Autodesk Inventor part; units mm, degrees
(part 3 of 4)
  line L1789 (3.9713, -18.6968) -> (3.9697, -18.8611)
  line L1790 (3.9697, -18.8611) -> (3.9623, -19.0574)
  line L1791 (3.9623, -19.0574) -> (3.944, -19.2862)
  line L1792 (3.944, -19.2862) -> (3.9122, -19.5462)
  line L1793 (3.9122, -19.5462) -> (3.8642, -19.8368)
  line L1794 (3.8642, -19.8368) -> (3.8334, -19.993)
  line L1795 (3.8334, -19.993) -> (3.7973, -20.1577)
  line L1796 (3.7973, -20.1577) -> (3.7564, -20.3275)
  line L1797 (3.7564, -20.3275) -> (3.709, -20.5077)
  line L1798 (3.709, -20.5077) -> (3.6602, -20.6786)
  arc A51 (2.909, -20.7975) -> (3.6602, -20.6786) centre (0, 0) ccw
  line L1799 (2.909, -20.7975) -> (2.8098, -20.6501)
  line L1800 (2.8098, -20.6501) -> (2.709, -20.4934)
  line L1801 (2.709, -20.4934) -> (2.6176, -20.3445)
  line L1802 (2.6176, -20.3445) -> (2.5324, -20.199)
  line L1803 (2.5324, -20.199) -> (2.4548, -20.06)
  line L1804 (2.4548, -20.06) -> (2.3194, -19.7984)
  line L1805 (2.3194, -19.7984) -> (2.2088, -19.561)
  line L1806 (2.2088, -19.561) -> (2.1207, -19.3491)
  line L1807 (2.1207, -19.3491) -> (2.0529, -19.1647)
  line L1808 (2.0529, -19.1647) -> (2.0007, -19.0089)
  line L1809 (2.0007, -19.0089) -> (1.9795, -18.9606)
  line L1810 (1.9795, -18.9606) -> (1.9573, -18.9216)
  line L1811 (1.9573, -18.9216) -> (1.9346, -18.8918)
  line L1812 (1.9346, -18.8918) -> (1.9116, -18.8713)
  line L1813 (1.9116, -18.8713) -> (1.8888, -18.86)
  line L1814 (1.8888, -18.86) -> (1.8665, -18.8579)
  line L1815 (1.8665, -18.8579) -> (1.833, -18.8612)
  line L1816 (1.833, -18.8612) -> (1.4868, -18.8916)
  line L1817 (1.4868, -18.8916) -> (1.1401, -18.9157)
  line L1818 (1.1401, -18.9157) -> (1.1065, -18.9177)
  line L1819 (1.1065, -18.9177) -> (1.0848, -18.9232)
  line L1820 (1.0848, -18.9232) -> (1.0641, -18.938)
  line L1821 (1.0641, -18.938) -> (1.0446, -18.9618)
  line L1822 (1.0446, -18.9618) -> (1.0268, -18.9948)
  line L1823 (1.0268, -18.9948) -> (1.011, -19.0369)
  line L1824 (1.011, -19.0369) -> (0.9976, -19.0878)
  line L1825 (0.9976, -19.0878) -> (0.9703, -19.2499)
  line L1826 (0.9703, -19.2499) -> (0.9323, -19.4427)
  line L1827 (0.9323, -19.4427) -> (0.8784, -19.6657)
  line L1828 (0.8784, -19.6657) -> (0.8063, -19.9175)
  line L1829 (0.8063, -19.9175) -> (0.7135, -20.1971)
  line L1830 (0.7135, -20.1971) -> (0.6586, -20.3465)
  line L1831 (0.6586, -20.3465) -> (0.5972, -20.5035)
  line L1832 (0.5972, -20.5035) -> (0.5302, -20.6649)
  line L1833 (0.5302, -20.6649) -> (0.4552, -20.8354)
  line L1834 (0.4552, -20.8354) -> (0.3803, -20.9966)
  arc A52 (-0.3803, -20.9966) -> (0.3803, -20.9966) centre (0, 0) ccw
  line L1835 (-0.3803, -20.9966) -> (-0.4552, -20.8354)
  line L1836 (-0.4552, -20.8354) -> (-0.5302, -20.6649)
  line L1837 (-0.5302, -20.6649) -> (-0.5972, -20.5035)
  line L1838 (-0.5972, -20.5035) -> (-0.6586, -20.3465)
  line L1839 (-0.6586, -20.3465) -> (-0.7135, -20.1971)
  line L1840 (-0.7135, -20.1971) -> (-0.8063, -19.9175)
  line L1841 (-0.8063, -19.9175) -> (-0.8784, -19.6657)
  line L1842 (-0.8784, -19.6657) -> (-0.9323, -19.4426)
  line L1843 (-0.9323, -19.4426) -> (-0.9703, -19.2499)
  line L1844 (-0.9703, -19.2499) -> (-0.9976, -19.0878)
  line L1845 (-0.9976, -19.0878) -> (-1.011, -19.0369)
  line L1846 (-1.011, -19.0369) -> (-1.0268, -18.9948)
  line L1847 (-1.0268, -18.9948) -> (-1.0446, -18.9618)
  line L1848 (-1.0446, -18.9618) -> (-1.0641, -18.938)
  line L1849 (-1.0641, -18.938) -> (-1.0848, -18.9232)
  line L1850 (-1.0848, -18.9232) -> (-1.1065, -18.9177)
  line L1851 (-1.1065, -18.9177) -> (-1.1401, -18.9157)
  line L1852 (-1.1401, -18.9157) -> (-1.4868, -18.8916)
  line L1853 (-1.4868, -18.8916) -> (-1.833, -18.8612)
  line L1854 (-1.833, -18.8612) -> (-1.8665, -18.8579)
  line L1855 (-1.8665, -18.8579) -> (-1.8888, -18.86)
  line L1856 (-1.8888, -18.86) -> (-1.9116, -18.8713)
  line L1857 (-1.9116, -18.8713) -> (-1.9346, -18.8918)
  line L1858 (-1.9346, -18.8918) -> (-1.9573, -18.9216)
  line L1859 (-1.9573, -18.9216) -> (-1.9795, -18.9606)
  line L1860 (-1.9795, -18.9606) -> (-2.0007, -19.0089)
  line L1861 (-2.0007, -19.0089) -> (-2.0529, -19.1647)
  line L1862 (-2.0529, -19.1647) -> (-2.1207, -19.3491)
  line L1863 (-2.1207, -19.3491) -> (-2.2088, -19.561)
  line L1864 (-2.2088, -19.561) -> (-2.3194, -19.7984)
  line L1865 (-2.3194, -19.7984) -> (-2.4548, -20.06)
  line L1866 (-2.4548, -20.06) -> (-2.5324, -20.199)
  line L1867 (-2.5324, -20.199) -> (-2.6176, -20.3445)
  line L1868 (-2.6176, -20.3445) -> (-2.709, -20.4934)
  line L1869 (-2.709, -20.4934) -> (-2.8098, -20.6501)
  line L1870 (-2.8098, -20.6501) -> (-2.909, -20.7975)
  arc A53 (-3.6602, -20.6786) -> (-2.909, -20.7975) centre (0, 0) ccw
  line L1871 (-3.6602, -20.6786) -> (-3.7089, -20.5077)
  line L1872 (-3.7089, -20.5077) -> (-3.7564, -20.3275)
  line L1873 (-3.7564, -20.3275) -> (-3.7973, -20.1577)
  line L1874 (-3.7973, -20.1577) -> (-3.8334, -19.993)
  line L1875 (-3.8334, -19.993) -> (-3.8642, -19.8368)
  line L1876 (-3.8642, -19.8368) -> (-3.9122, -19.5462)
  line L1877 (-3.9122, -19.5462) -> (-3.944, -19.2862)
  line L1878 (-3.944, -19.2862) -> (-3.9623, -19.0574)
  line L1879 (-3.9623, -19.0574) -> (-3.9697, -18.8611)
  line L1880 (-3.9697, -18.8611) -> (-3.9713, -18.6968)
  line L1881 (-3.9713, -18.6968) -> (-3.9765, -18.6443)
  line L1882 (-3.9765, -18.6443) -> (-3.9856, -18.6004)
  line L1883 (-3.9856, -18.6004) -> (-3.998, -18.565)
  line L1884 (-3.998, -18.565) -> (-4.0135, -18.5383)
  line L1885 (-4.0135, -18.5383) -> (-4.0317, -18.5206)
  line L1886 (-4.0317, -18.5206) -> (-4.0522, -18.5117)
  line L1887 (-4.0522, -18.5117) -> (-4.0852, -18.5045)
  line L1888 (-4.0852, -18.5045) -> (-4.4238, -18.4264)
  line L1889 (-4.4238, -18.4264) -> (-4.761, -18.3423)
  line L1890 (-4.761, -18.3423) -> (-4.7936, -18.3337)
  line L1891 (-4.7936, -18.3337) -> (-4.8159, -18.3323)
  line L1892 (-4.8159, -18.3323) -> (-4.8402, -18.3399)
  line L1893 (-4.8402, -18.3399) -> (-4.8661, -18.3566)
  line L1894 (-4.8661, -18.3566) -> (-4.8932, -18.3825)
  line L1895 (-4.8932, -18.3825) -> (-4.9212, -18.4175)
  line L1896 (-4.9212, -18.4175) -> (-4.9497, -18.4619)
  line L1897 (-4.9497, -18.4619) -> (-5.0257, -18.6076)
  line L1898 (-5.0257, -18.6076) -> (-5.1215, -18.7791)
  line L1899 (-5.1215, -18.7791) -> (-5.2416, -18.9746)
  line L1900 (-5.2416, -18.9746) -> (-5.388, -19.1919)
  line L1901 (-5.388, -19.1919) -> (-5.5627, -19.429)
  line L1902 (-5.5627, -19.429) -> (-5.661, -19.5542)
  line L1903 (-5.661, -19.5542) -> (-5.7679, -19.6846)
  line L1904 (-5.7679, -19.6846) -> (-5.8815, -19.8173)
  line L1905 (-5.8815, -19.8173) -> (-6.0056, -19.9563)
  line L1906 (-6.0056, -19.9563) -> (-6.1266, -20.0864)
  arc A54 (-6.85, -19.8514) -> (-6.1266, -20.0864) centre (0, 0) ccw
  line L1907 (-6.85, -19.8514) -> (-6.8714, -19.675)
  line L1908 (-6.8714, -19.675) -> (-6.8901, -19.4896)
  line L1909 (-6.8901, -19.4896) -> (-6.9039, -19.3155)
  line L1910 (-6.9039, -19.3155) -> (-6.9138, -19.1472)
  line L1911 (-6.9138, -19.1472) -> (-6.9198, -18.9881)
  line L1912 (-6.9198, -18.9881) -> (-6.9217, -18.6935)
  line L1913 (-6.9217, -18.6935) -> (-6.9124, -18.4318)
  line L1914 (-6.9124, -18.4318) -> (-6.8947, -18.203)
  line L1915 (-6.8947, -18.203) -> (-6.8714, -18.0079)
  line L1916 (-6.8714, -18.0079) -> (-6.8472, -17.8454)
  line L1917 (-6.8472, -17.8454) -> (-6.8442, -17.7927)
  line L1918 (-6.8442, -17.7927) -> (-6.8462, -17.7479)
  line L1919 (-6.8462, -17.7479) -> (-6.853, -17.711)
  line L1920 (-6.853, -17.711) -> (-6.8641, -17.6823)
  line L1921 (-6.8641, -17.6823) -> (-6.8793, -17.6618)
  line L1922 (-6.8793, -17.6618) -> (-6.8982, -17.6499)
  line L1923 (-6.8982, -17.6499) -> (-6.9296, -17.6376)
  line L1924 (-6.9296, -17.6376) -> (-7.2519, -17.5075)
  line L1925 (-7.2519, -17.5075) -> (-7.5717, -17.3717)
  line L1926 (-7.5717, -17.3717) -> (-7.6026, -17.3581)
  line L1927 (-7.6026, -17.3581) -> (-7.6244, -17.3532)
  line L1928 (-7.6244, -17.3532) -> (-7.6496, -17.3569)
  line L1929 (-7.6496, -17.3569) -> (-7.6778, -17.3694)
  line L1930 (-7.6778, -17.3694) -> (-7.7086, -17.3907)
  line L1931 (-7.7086, -17.3907) -> (-7.7418, -17.4209)
  line L1932 (-7.7418, -17.4209) -> (-7.7769, -17.4603)
  line L1933 (-7.7769, -17.4603) -> (-7.8747, -17.5923)
  line L1934 (-7.8747, -17.5923) -> (-7.9961, -17.7468)
  line L1935 (-7.9961, -17.7468) -> (-8.1454, -17.9211)
  line L1936 (-8.1454, -17.9211) -> (-8.3239, -18.1127)
  line L1937 (-8.3239, -18.1127) -> (-8.5336, -18.3196)
  line L1938 (-8.5336, -18.3196) -> (-8.6503, -18.4279)
  line L1939 (-8.6503, -18.4279) -> (-8.7763, -18.5399)
  line L1940 (-8.7763, -18.5399) -> (-8.9092, -18.6532)
  line L1941 (-8.9092, -18.6532) -> (-9.0535, -18.7712)
  line L1942 (-9.0535, -18.7712) -> (-9.1934, -18.8807)
  arc A55 (-9.8711, -18.5354) -> (-9.1934, -18.8807) centre (0, 0) ccw
  line L1943 (-9.8711, -18.5354) -> (-9.8647, -18.3579)
  line L1944 (-9.8647, -18.3579) -> (-9.8541, -18.1718)
  line L1945 (-9.8541, -18.1718) -> (-9.8405, -17.9977)
  line L1946 (-9.8405, -17.9977) -> (-9.8239, -17.8299)
  line L1947 (-9.8239, -17.8299) -> (-9.805, -17.6718)
  line L1948 (-9.805, -17.6718) -> (-9.7608, -17.3806)
  line L1949 (-9.7608, -17.3806) -> (-9.7107, -17.1235)
  line L1950 (-9.7107, -17.1235) -> (-9.6574, -16.9003)
  line L1951 (-9.6574, -16.9003) -> (-9.6038, -16.7112)
  line L1952 (-9.6038, -16.7112) -> (-9.5545, -16.5545)
  line L1953 (-9.5545, -16.5545) -> (-9.5433, -16.503)
  line L1954 (-9.5433, -16.503) -> (-9.5383, -16.4584)
  line L1955 (-9.5383, -16.4584) -> (-9.5392, -16.4209)
  line L1956 (-9.5392, -16.4209) -> (-9.5457, -16.3908)
  line L1957 (-9.5457, -16.3908) -> (-9.5575, -16.3682)
  line L1958 (-9.5575, -16.3682) -> (-9.5743, -16.3535)
  line L1959 (-9.5743, -16.3535) -> (-9.6034, -16.3365)
  line L1960 (-9.6034, -16.3365) -> (-9.9013, -16.1575)
  line L1961 (-9.9013, -16.1575) -> (-10.196, -15.9733)
  line L1962 (-10.196, -15.9733) -> (-10.2244, -15.9551)
  line L1963 (-10.2244, -15.9551) -> (-10.2452, -15.9469)
  line L1964 (-10.2452, -15.9469) -> (-10.2706, -15.9466)
  line L1965 (-10.2706, -15.9466) -> (-10.3004, -15.9544)
  line L1966 (-10.3004, -15.9544) -> (-10.3342, -15.9707)
  line L1967 (-10.3342, -15.9707) -> (-10.3717, -15.9954)
  line L1968 (-10.3717, -15.9954) -> (-10.4125, -16.0287)
  line L1969 (-10.4125, -16.0287) -> (-10.5298, -16.1438)
  line L1970 (-10.5298, -16.1438) -> (-10.6739, -16.2774)
  line L1971 (-10.6739, -16.2774) -> (-10.8486, -16.4262)
  line L1972 (-10.8486, -16.4262) -> (-11.0549, -16.5875)
  line L1973 (-11.0549, -16.5875) -> (-11.2943, -16.7591)
  line L1974 (-11.2943, -16.7591) -> (-11.4265, -16.8478)
  line L1975 (-11.4265, -16.8478) -> (-11.5685, -16.9387)
  line L1976 (-11.5685, -16.9387) -> (-11.7175, -17.0299)
  line L1977 (-11.7175, -17.0299) -> (-11.8785, -17.1238)
  line L1978 (-11.8785, -17.1238) -> (-12.0338, -17.2101)
  arc A56 (-12.6491, -16.7631) -> (-12.0338, -17.2101) centre (0, 0) ccw
  line L1979 (-12.6491, -16.7631) -> (-12.615, -16.5887)
  line L1980 (-12.615, -16.5887) -> (-12.5755, -16.4066)
  line L1981 (-12.5755, -16.4066) -> (-12.5348, -16.2367)
  line L1982 (-12.5348, -16.2367) -> (-12.4922, -16.0736)
  line L1983 (-12.4922, -16.0736) -> (-12.4487, -15.9204)
  line L1984 (-12.4487, -15.9204) -> (-12.3595, -15.6397)
  line L1985 (-12.3595, -15.6397) -> (-12.2698, -15.3936)
  line L1986 (-12.2698, -15.3936) -> (-12.1823, -15.1815)
  line L1987 (-12.1823, -15.1815) -> (-12.0998, -15.0031)
  line L1988 (-12.0998, -15.0031) -> (-12.0266, -14.856)
  line L1989 (-12.0266, -14.856) -> (-12.0075, -14.8069)
  line L1990 (-12.0075, -14.8069) -> (-11.9956, -14.7636)
  line L1991 (-11.9956, -14.7636) -> (-11.9906, -14.7265)
  line L1992 (-11.9906, -14.7265) -> (-11.9923, -14.6957)
  line L1993 (-11.9923, -14.6957) -> (-12.0004, -14.6716)
  line L1994 (-12.0004, -14.6716) -> (-12.0147, -14.6544)
  line L1995 (-12.0147, -14.6544) -> (-12.0408, -14.633)
  line L1996 (-12.0408, -14.633) -> (-12.307, -14.4097)
  line L1997 (-12.307, -14.4097) -> (-12.5693, -14.1816)
  line L1998 (-12.5693, -14.1816) -> (-12.5944, -14.1592)
  line L1999 (-12.5944, -14.1592) -> (-12.6137, -14.1478)
  line L2000 (-12.6137, -14.1478) -> (-12.6387, -14.1436)
  line L2001 (-12.6387, -14.1436) -> (-12.6694, -14.1467)
  line L2002 (-12.6694, -14.1467) -> (-12.7053, -14.1574)
  line L2003 (-12.7053, -14.1574) -> (-12.7462, -14.176)
  line L2004 (-12.7462, -14.176) -> (-12.7918, -14.2025)
  line L2005 (-12.7918, -14.2025) -> (-12.9256, -14.2978)
  line L2006 (-12.9256, -14.2978) -> (-13.0888, -14.4072)
  line L2007 (-13.0888, -14.4072) -> (-13.2846, -14.5269)
  line L2008 (-13.2846, -14.5269) -> (-13.5137, -14.654)
  line L2009 (-13.5137, -14.654) -> (-13.777, -14.786)
  line L2010 (-13.777, -14.786) -> (-13.9214, -14.8529)
  line L2011 (-13.9214, -14.8529) -> (-14.0759, -14.9205)
  line L2012 (-14.0759, -14.9205) -> (-14.2373, -14.9872)
  line L2013 (-14.2373, -14.9872) -> (-14.411, -15.0547)
  line L2014 (-14.411, -15.0547) -> (-14.5779, -15.1157)
  arc A57 (-15.1157, -14.5779) -> (-14.5779, -15.1157) centre (0, 0) ccw
  line L2015 (-15.1157, -14.5779) -> (-15.0547, -14.411)
  line L2016 (-15.0547, -14.411) -> (-14.9872, -14.2373)
  line L2017 (-14.9872, -14.2373) -> (-14.9205, -14.0759)
  line L2018 (-14.9205, -14.0759) -> (-14.8529, -13.9214)
  line L2019 (-14.8529, -13.9214) -> (-14.786, -13.777)
  line L2020 (-14.786, -13.777) -> (-14.654, -13.5137)
  line L2021 (-14.654, -13.5137) -> (-14.5269, -13.2846)
  line L2022 (-14.5269, -13.2846) -> (-14.4072, -13.0888)
  line L2023 (-14.4072, -13.0888) -> (-14.2978, -12.9256)
  line L2024 (-14.2978, -12.9256) -> (-14.2025, -12.7918)
  line L2025 (-14.2025, -12.7918) -> (-14.1759, -12.7462)
  line L2026 (-14.1759, -12.7462) -> (-14.1574, -12.7053)
  line L2027 (-14.1574, -12.7053) -> (-14.1467, -12.6694)
  line L2028 (-14.1467, -12.6694) -> (-14.1436, -12.6388)
  line L2029 (-14.1436, -12.6388) -> (-14.1478, -12.6137)
  line L2030 (-14.1478, -12.6137) -> (-14.1592, -12.5944)
  line L2031 (-14.1592, -12.5944) -> (-14.1816, -12.5693)
  line L2032 (-14.1816, -12.5693) -> (-14.4097, -12.307)
  line L2033 (-14.4097, -12.307) -> (-14.633, -12.0408)
  line L2034 (-14.633, -12.0408) -> (-14.6544, -12.0147)
  line L2035 (-14.6544, -12.0147) -> (-14.6716, -12.0004)
  line L2036 (-14.6716, -12.0004) -> (-14.6957, -11.9923)
  line L2037 (-14.6957, -11.9923) -> (-14.7265, -11.9906)
  line L2038 (-14.7265, -11.9906) -> (-14.7636, -11.9956)
  line L2039 (-14.7636, -11.9956) -> (-14.8069, -12.0075)
  line L2040 (-14.8069, -12.0075) -> (-14.856, -12.0266)
  line L2041 (-14.856, -12.0266) -> (-15.0031, -12.0998)
  line L2042 (-15.0031, -12.0998) -> (-15.1815, -12.1823)
  line L2043 (-15.1815, -12.1823) -> (-15.3936, -12.2699)
  line L2044 (-15.3936, -12.2699) -> (-15.6397, -12.3595)
  line L2045 (-15.6397, -12.3595) -> (-15.9204, -12.4487)
  line L2046 (-15.9204, -12.4487) -> (-16.0735, -12.4922)
  line L2047 (-16.0735, -12.4922) -> (-16.2367, -12.5348)
  line L2048 (-16.2367, -12.5348) -> (-16.4066, -12.5755)
  line L2049 (-16.4066, -12.5755) -> (-16.5887, -12.615)
  line L2050 (-16.5887, -12.615) -> (-16.763, -12.6491)
  arc A58 (-17.2101, -12.0338) -> (-16.763, -12.6491) centre (0, 0) ccw
  line L2051 (-17.2101, -12.0338) -> (-17.1238, -11.8785)
  line L2052 (-17.1238, -11.8785) -> (-17.0299, -11.7175)
  line L2053 (-17.0299, -11.7175) -> (-16.9387, -11.5685)
  line L2054 (-16.9387, -11.5685) -> (-16.8478, -11.4266)
  line L2055 (-16.8478, -11.4266) -> (-16.7591, -11.2943)
  line L2056 (-16.7591, -11.2943) -> (-16.5875, -11.0549)
  line L2057 (-16.5875, -11.0549) -> (-16.4262, -10.8486)
  line L2058 (-16.4262, -10.8486) -> (-16.2774, -10.6739)
  line L2059 (-16.2774, -10.6739) -> (-16.1438, -10.5298)
  line L2060 (-16.1438, -10.5298) -> (-16.0287, -10.4125)
  line L2061 (-16.0287, -10.4125) -> (-15.9954, -10.3717)
  line L2062 (-15.9954, -10.3717) -> (-15.9707, -10.3342)
  line L2063 (-15.9707, -10.3342) -> (-15.9544, -10.3004)
  line L2064 (-15.9544, -10.3004) -> (-15.9466, -10.2706)
  line L2065 (-15.9466, -10.2706) -> (-15.9468, -10.2452)
  line L2066 (-15.9468, -10.2452) -> (-15.9551, -10.2244)
  line L2067 (-15.9551, -10.2244) -> (-15.9733, -10.196)
  line L2068 (-15.9733, -10.196) -> (-16.1575, -9.9014)
  line L2069 (-16.1575, -9.9014) -> (-16.3364, -9.6034)
  line L2070 (-16.3364, -9.6034) -> (-16.3534, -9.5743)
  line L2071 (-16.3534, -9.5743) -> (-16.3682, -9.5575)
  line L2072 (-16.3682, -9.5575) -> (-16.3908, -9.5457)
  line L2073 (-16.3908, -9.5457) -> (-16.4209, -9.5392)
  line L2074 (-16.4209, -9.5392) -> (-16.4584, -9.5383)
  line L2075 (-16.4584, -9.5383) -> (-16.503, -9.5433)
  line L2076 (-16.503, -9.5433) -> (-16.5545, -9.5545)
  line L2077 (-16.5545, -9.5545) -> (-16.7112, -9.6038)
  line L2078 (-16.7112, -9.6038) -> (-16.9003, -9.6574)
  line L2079 (-16.9003, -9.6574) -> (-17.1235, -9.7107)
  line L2080 (-17.1235, -9.7107) -> (-17.3806, -9.7608)
  line L2081 (-17.3806, -9.7608) -> (-17.6718, -9.805)
  line L2082 (-17.6718, -9.805) -> (-17.8299, -9.8239)
  line L2083 (-17.8299, -9.8239) -> (-17.9976, -9.8405)
  line L2084 (-17.9976, -9.8405) -> (-18.1718, -9.8541)
  line L2085 (-18.1718, -9.8541) -> (-18.3579, -9.8647)
  line L2086 (-18.3579, -9.8647) -> (-18.5354, -9.8711)
  arc A59 (-18.8807, -9.1934) -> (-18.5354, -9.8711) centre (0, 0) ccw
  line L2087 (-18.8807, -9.1934) -> (-18.7712, -9.0535)
  line L2088 (-18.7712, -9.0535) -> (-18.6532, -8.9092)
  line L2089 (-18.6532, -8.9092) -> (-18.5399, -8.7763)
  line L2090 (-18.5399, -8.7763) -> (-18.4279, -8.6503)
  line L2091 (-18.4279, -8.6503) -> (-18.3196, -8.5336)
  line L2092 (-18.3196, -8.5336) -> (-18.1127, -8.324)
  line L2093 (-18.1127, -8.324) -> (-17.9211, -8.1454)
  line L2094 (-17.9211, -8.1454) -> (-17.7468, -7.9961)
  line L2095 (-17.7468, -7.9961) -> (-17.5923, -7.8747)
  line L2096 (-17.5923, -7.8747) -> (-17.4603, -7.7769)
  line L2097 (-17.4603, -7.7769) -> (-17.4209, -7.7418)
  line L2098 (-17.4209, -7.7418) -> (-17.3907, -7.7086)
  line L2099 (-17.3907, -7.7086) -> (-17.3694, -7.6778)
  line L2100 (-17.3694, -7.6778) -> (-17.3569, -7.6496)
  line L2101 (-17.3569, -7.6496) -> (-17.3532, -7.6244)
  line L2102 (-17.3532, -7.6244) -> (-17.3581, -7.6026)
  line L2103 (-17.3581, -7.6026) -> (-17.3717, -7.5717)
  line L2104 (-17.3717, -7.5717) -> (-17.5075, -7.2519)
  line L2105 (-17.5075, -7.2519) -> (-17.6376, -6.9296)
  line L2106 (-17.6376, -6.9296) -> (-17.6499, -6.8982)
  line L2107 (-17.6499, -6.8982) -> (-17.6618, -6.8793)
  line L2108 (-17.6618, -6.8793) -> (-17.6823, -6.8641)
  line L2109 (-17.6823, -6.8641) -> (-17.711, -6.853)
  line L2110 (-17.711, -6.853) -> (-17.7479, -6.8462)
  line L2111 (-17.7479, -6.8462) -> (-17.7927, -6.8442)
  line L2112 (-17.7927, -6.8442) -> (-17.8453, -6.8472)
  line L2113 (-17.8453, -6.8472) -> (-18.0079, -6.8714)
  line L2114 (-18.0079, -6.8714) -> (-18.203, -6.8948)
  line L2115 (-18.203, -6.8948) -> (-18.4318, -6.9124)
  line L2116 (-18.4318, -6.9124) -> (-18.6935, -6.9217)
  line L2117 (-18.6935, -6.9217) -> (-18.9881, -6.9198)
  line L2118 (-18.9881, -6.9198) -> (-19.1471, -6.9138)
  line L2119 (-19.1471, -6.9138) -> (-19.3155, -6.9039)
  line L2120 (-19.3155, -6.9039) -> (-19.4896, -6.8901)
  line L2121 (-19.4896, -6.8901) -> (-19.675, -6.8714)
  line L2122 (-19.675, -6.8714) -> (-19.8514, -6.85)
  arc A60 (-20.0864, -6.1266) -> (-19.8514, -6.85) centre (0, 0) ccw
  line L2123 (-20.0864, -6.1266) -> (-19.9563, -6.0056)
  line L2124 (-19.9563, -6.0056) -> (-19.8173, -5.8815)
  line L2125 (-19.8173, -5.8815) -> (-19.6846, -5.768)
  line L2126 (-19.6846, -5.768) -> (-19.5542, -5.661)
  line L2127 (-19.5542, -5.661) -> (-19.429, -5.5627)
  line L2128 (-19.429, -5.5627) -> (-19.1918, -5.388)
  line L2129 (-19.1918, -5.388) -> (-18.9746, -5.2416)
  line L2130 (-18.9746, -5.2416) -> (-18.7791, -5.1215)
  line L2131 (-18.7791, -5.1215) -> (-18.6076, -5.0257)
  line L2132 (-18.6076, -5.0257) -> (-18.4619, -4.9497)
  line L2133 (-18.4619, -4.9497) -> (-18.4175, -4.9212)
  line L2134 (-18.4175, -4.9212) -> (-18.3824, -4.8932)
  line L2135 (-18.3824, -4.8932) -> (-18.3566, -4.8661)
  line L2136 (-18.3566, -4.8661) -> (-18.3399, -4.8402)
  line L2137 (-18.3399, -4.8402) -> (-18.3323, -4.8159)
  line L2138 (-18.3323, -4.8159) -> (-18.3337, -4.7936)
  line L2139 (-18.3337, -4.7936) -> (-18.3423, -4.761)
  line L2140 (-18.3423, -4.761) -> (-18.4264, -4.4238)
  line L2141 (-18.4264, -4.4238) -> (-18.5045, -4.0852)
  line L2142 (-18.5045, -4.0852) -> (-18.5117, -4.0522)
  line L2143 (-18.5117, -4.0522) -> (-18.5205, -4.0317)
  line L2144 (-18.5205, -4.0317) -> (-18.5383, -4.0135)
  line L2145 (-18.5383, -4.0135) -> (-18.565, -3.998)
  line L2146 (-18.565, -3.998) -> (-18.6003, -3.9856)
  line L2147 (-18.6003, -3.9856) -> (-18.6443, -3.9765)
  line L2148 (-18.6443, -3.9765) -> (-18.6968, -3.9713)
  line L2149 (-18.6968, -3.9713) -> (-18.8611, -3.9697)
  line L2150 (-18.8611, -3.9697) -> (-19.0574, -3.9623)
  line L2151 (-19.0574, -3.9623) -> (-19.2862, -3.944)
  line L2152 (-19.2862, -3.944) -> (-19.5462, -3.9122)
  line L2153 (-19.5462, -3.9122) -> (-19.8368, -3.8642)
  line L2154 (-19.8368, -3.8642) -> (-19.993, -3.8334)
  line L2155 (-19.993, -3.8334) -> (-20.1577, -3.7973)
  line L2156 (-20.1577, -3.7973) -> (-20.3275, -3.7564)
  line L2157 (-20.3275, -3.7564) -> (-20.5077, -3.709)
  line L2158 (-20.5077, -3.709) -> (-20.6786, -3.6602)
  arc A61 (-20.7975, -2.909) -> (-20.6786, -3.6602) centre (0, 0) ccw
  line L2159 (-20.7975, -2.909) -> (-20.6501, -2.8098)
  line L2160 (-20.6501, -2.8098) -> (-20.4934, -2.709)
  line L2161 (-20.4934, -2.709) -> (-20.3445, -2.6176)
  line L2162 (-20.3445, -2.6176) -> (-20.199, -2.5324)
  line L2163 (-20.199, -2.5324) -> (-20.06, -2.4549)
  line L2164 (-20.06, -2.4549) -> (-19.7984, -2.3194)
  line L2165 (-19.7984, -2.3194) -> (-19.561, -2.2088)
  line L2166 (-19.561, -2.2088) -> (-19.3491, -2.1207)
  line L2167 (-19.3491, -2.1207) -> (-19.1647, -2.053)
  line L2168 (-19.1647, -2.053) -> (-19.0089, -2.0007)
  line L2169 (-19.0089, -2.0007) -> (-18.9606, -1.9795)
  line L2170 (-18.9606, -1.9795) -> (-18.9216, -1.9573)
  line L2171 (-18.9216, -1.9573) -> (-18.8918, -1.9346)
  line L2172 (-18.8918, -1.9346) -> (-18.8713, -1.9116)
  line L2173 (-18.8713, -1.9116) -> (-18.8599, -1.8888)
  line L2174 (-18.8599, -1.8888) -> (-18.8579, -1.8665)
  line L2175 (-18.8579, -1.8665) -> (-18.8612, -1.833)
  line L2176 (-18.8612, -1.833) -> (-18.8916, -1.4868)
  line L2177 (-18.8916, -1.4868) -> (-18.9157, -1.1401)
  line L2178 (-18.9157, -1.1401) -> (-18.9177, -1.1065)
  line L2179 (-18.9177, -1.1065) -> (-18.9232, -1.0848)
  line L2180 (-18.9232, -1.0848) -> (-18.938, -1.0641)
  line L2181 (-18.938, -1.0641) -> (-18.9618, -1.0446)
  line L2182 (-18.9618, -1.0446) -> (-18.9948, -1.0268)
  line L2183 (-18.9948, -1.0268) -> (-19.0368, -1.011)
  line L2184 (-19.0368, -1.011) -> (-19.0878, -0.9976)
  line L2185 (-19.0878, -0.9976) -> (-19.2499, -0.9703)
  line L2186 (-19.2499, -0.9703) -> (-19.4426, -0.9323)
  line L2187 (-19.4426, -0.9323) -> (-19.6657, -0.8784)
  line L2188 (-19.6657, -0.8784) -> (-19.9175, -0.8063)
  line L2189 (-19.9175, -0.8063) -> (-20.1971, -0.7135)
  line L2190 (-20.1971, -0.7135) -> (-20.3465, -0.6586)
  line L2191 (-20.3465, -0.6586) -> (-20.5035, -0.5972)
  line L2192 (-20.5035, -0.5972) -> (-20.6649, -0.5302)
  line L2193 (-20.6649, -0.5302) -> (-20.8354, -0.4552)
  line L2194 (-20.8354, -0.4552) -> (-20.9966, -0.3803)
  arc A62 (-20.9966, 0.3803) -> (-20.9966, -0.3803) centre (0, 0) ccw
  line L2195 (-20.9966, 0.3803) -> (-20.8354, 0.4552)
  line L2196 (-20.8354, 0.4552) -> (-20.6649, 0.5302)
  line L2197 (-20.6649, 0.5302) -> (-20.5035, 0.5972)
  line L2198 (-20.5035, 0.5972) -> (-20.3465, 0.6586)
  line L2199 (-20.3465, 0.6586) -> (-20.1971, 0.7134)
  line L2200 (-20.1971, 0.7134) -> (-19.9175, 0.8063)
  line L2201 (-19.9175, 0.8063) -> (-19.6657, 0.8784)
  line L2202 (-19.6657, 0.8784) -> (-19.4426, 0.9323)
  line L2203 (-19.4426, 0.9323) -> (-19.2499, 0.9703)
  line L2204 (-19.2499, 0.9703) -> (-19.0878, 0.9976)
  line L2205 (-19.0878, 0.9976) -> (-19.0368, 1.011)
  line L2206 (-19.0368, 1.011) -> (-18.9948, 1.0268)
  line L2207 (-18.9948, 1.0268) -> (-18.9618, 1.0446)
  line L2208 (-18.9618, 1.0446) -> (-18.938, 1.0641)
  line L2209 (-18.938, 1.0641) -> (-18.9232, 1.0848)
  line L2210 (-18.9232, 1.0848) -> (-18.9177, 1.1065)
  line L2211 (-18.9177, 1.1065) -> (-18.9157, 1.1401)
  line L2212 (-18.9157, 1.1401) -> (-18.8916, 1.4868)
  line L2213 (-18.8916, 1.4868) -> (-18.8612, 1.833)
  line L2214 (-18.8612, 1.833) -> (-18.8579, 1.8665)
  line L2215 (-18.8579, 1.8665) -> (-18.8599, 1.8888)
  line L2216 (-18.8599, 1.8888) -> (-18.8713, 1.9116)
  line L2217 (-18.8713, 1.9116) -> (-18.8918, 1.9346)
  line L2218 (-18.8918, 1.9346) -> (-18.9216, 1.9573)
  line L2219 (-18.9216, 1.9573) -> (-18.9606, 1.9795)
  line L2220 (-18.9606, 1.9795) -> (-19.0089, 2.0007)
  line L2221 (-19.0089, 2.0007) -> (-19.1647, 2.0529)
  line L2222 (-19.1647, 2.0529) -> (-19.3491, 2.1207)
  line L2223 (-19.3491, 2.1207) -> (-19.561, 2.2088)
  line L2224 (-19.561, 2.2088) -> (-19.7984, 2.3194)
  line L2225 (-19.7984, 2.3194) -> (-20.06, 2.4548)
  line L2226 (-20.06, 2.4548) -> (-20.199, 2.5324)
  line L2227 (-20.199, 2.5324) -> (-20.3445, 2.6176)
  line L2228 (-20.3445, 2.6176) -> (-20.4934, 2.709)
  line L2229 (-20.4934, 2.709) -> (-20.6501, 2.8098)
  line L2230 (-20.6501, 2.8098) -> (-20.7975, 2.909)
  arc A63 (-20.6786, 3.6602) -> (-20.7975, 2.909) centre (0, 0) ccw
  line L2231 (-20.6786, 3.6602) -> (-20.5077, 3.7089)
  line L2232 (-20.5077, 3.7089) -> (-20.3275, 3.7564)
  line L2233 (-20.3275, 3.7564) -> (-20.1577, 3.7973)
  line L2234 (-20.1577, 3.7973) -> (-19.993, 3.8334)
  line L2235 (-19.993, 3.8334) -> (-19.8368, 3.8642)
  line L2236 (-19.8368, 3.8642) -> (-19.5462, 3.9121)
  line L2237 (-19.5462, 3.9121) -> (-19.2862, 3.944)
  line L2238 (-19.2862, 3.944) -> (-19.0574, 3.9623)
  line L2239 (-19.0574, 3.9623) -> (-18.8611, 3.9697)
  line L2240 (-18.8611, 3.9697) -> (-18.6968, 3.9713)
  line L2241 (-18.6968, 3.9713) -> (-18.6443, 3.9765)
  line L2242 (-18.6443, 3.9765) -> (-18.6003, 3.9856)
  line L2243 (-18.6003, 3.9856) -> (-18.565, 3.998)
  line L2244 (-18.565, 3.998) -> (-18.5383, 4.0135)
  line L2245 (-18.5383, 4.0135) -> (-18.5205, 4.0317)
  line L2246 (-18.5205, 4.0317) -> (-18.5117, 4.0522)
  line L2247 (-18.5117, 4.0522) -> (-18.5045, 4.0851)
  line L2248 (-18.5045, 4.0851) -> (-18.4264, 4.4238)
  line L2249 (-18.4264, 4.4238) -> (-18.3423, 4.761)
  line L2250 (-18.3423, 4.761) -> (-18.3337, 4.7936)
  line L2251 (-18.3337, 4.7936) -> (-18.3323, 4.8159)
  line L2252 (-18.3323, 4.8159) -> (-18.3399, 4.8402)
  line L2253 (-18.3399, 4.8402) -> (-18.3566, 4.8661)
  line L2254 (-18.3566, 4.8661) -> (-18.3824, 4.8932)
  line L2255 (-18.3824, 4.8932) -> (-18.4175, 4.9212)
  line L2256 (-18.4175, 4.9212) -> (-18.4619, 4.9497)
  line L2257 (-18.4619, 4.9497) -> (-18.6076, 5.0257)
  line L2258 (-18.6076, 5.0257) -> (-18.7791, 5.1215)
  line L2259 (-18.7791, 5.1215) -> (-18.9746, 5.2416)
  line L2260 (-18.9746, 5.2416) -> (-19.1918, 5.388)
  line L2261 (-19.1918, 5.388) -> (-19.429, 5.5627)
  line L2262 (-19.429, 5.5627) -> (-19.5542, 5.661)
  line L2263 (-19.5542, 5.661) -> (-19.6846, 5.7679)
  line L2264 (-19.6846, 5.7679) -> (-19.8173, 5.8815)
  line L2265 (-19.8173, 5.8815) -> (-19.9563, 6.0056)
  line L2266 (-19.9563, 6.0056) -> (-20.0864, 6.1266)
  arc A64 (-19.8514, 6.85) -> (-20.0864, 6.1266) centre (0, 0) ccw
  line L2267 (-19.8514, 6.85) -> (-19.675, 6.8714)
  line L2268 (-19.675, 6.8714) -> (-19.4896, 6.8901)
  line L2269 (-19.4896, 6.8901) -> (-19.3155, 6.9039)
  line L2270 (-19.3155, 6.9039) -> (-19.1471, 6.9138)
  line L2271 (-19.1471, 6.9138) -> (-18.9881, 6.9198)
  line L2272 (-18.9881, 6.9198) -> (-18.6935, 6.9217)
  line L2273 (-18.6935, 6.9217) -> (-18.4318, 6.9124)
  line L2274 (-18.4318, 6.9124) -> (-18.203, 6.8947)
  line L2275 (-18.203, 6.8947) -> (-18.0079, 6.8714)
  line L2276 (-18.0079, 6.8714) -> (-17.8453, 6.8472)
  line L2277 (-17.8453, 6.8472) -> (-17.7927, 6.8442)
  line L2278 (-17.7927, 6.8442) -> (-17.7479, 6.8462)
  line L2279 (-17.7479, 6.8462) -> (-17.711, 6.853)
  line L2280 (-17.711, 6.853) -> (-17.6823, 6.8641)
  line L2281 (-17.6823, 6.8641) -> (-17.6618, 6.8793)
  line L2282 (-17.6618, 6.8793) -> (-17.6499, 6.8982)
  line L2283 (-17.6499, 6.8982) -> (-17.6376, 6.9296)
  line L2284 (-17.6376, 6.9296) -> (-17.5075, 7.2518)
  line L2285 (-17.5075, 7.2518) -> (-17.3716, 7.5717)
  line L2286 (-17.3716, 7.5717) -> (-17.3581, 7.6026)
  line L2287 (-17.3581, 7.6026) -> (-17.3532, 7.6244)
  line L2288 (-17.3532, 7.6244) -> (-17.3569, 7.6496)
  line L2289 (-17.3569, 7.6496) -> (-17.3694, 7.6778)
  line L2290 (-17.3694, 7.6778) -> (-17.3907, 7.7086)
  line L2291 (-17.3907, 7.7086) -> (-17.4209, 7.7418)
  line L2292 (-17.4209, 7.7418) -> (-17.4603, 7.7769)
  line L2293 (-17.4603, 7.7769) -> (-17.5923, 7.8747)
  line L2294 (-17.5923, 7.8747) -> (-17.7468, 7.9961)
  line L2295 (-17.7468, 7.9961) -> (-17.9211, 8.1454)
  line L2296 (-17.9211, 8.1454) -> (-18.1127, 8.3239)
  line L2297 (-18.1127, 8.3239) -> (-18.3196, 8.5336)
  line L2298 (-18.3196, 8.5336) -> (-18.4279, 8.6503)
  line L2299 (-18.4279, 8.6503) -> (-18.5399, 8.7763)
  line L2300 (-18.5399, 8.7763) -> (-18.6532, 8.9092)
  line L2301 (-18.6532, 8.9092) -> (-18.7712, 9.0535)
  line L2302 (-18.7712, 9.0535) -> (-18.8807, 9.1934)
  arc A65 (-18.5354, 9.8711) -> (-18.8807, 9.1934) centre (0, 0) ccw
  line L2303 (-18.5354, 9.8711) -> (-18.3579, 9.8646)
  line L2304 (-18.3579, 9.8646) -> (-18.1718, 9.8541)
  line L2305 (-18.1718, 9.8541) -> (-17.9976, 9.8405)
  line L2306 (-17.9976, 9.8405) -> (-17.8299, 9.8239)
  line L2307 (-17.8299, 9.8239) -> (-17.6718, 9.805)
  line L2308 (-17.6718, 9.805) -> (-17.3806, 9.7608)
  line L2309 (-17.3806, 9.7608) -> (-17.1235, 9.7107)
  line L2310 (-17.1235, 9.7107) -> (-16.9003, 9.6574)
  line L2311 (-16.9003, 9.6574) -> (-16.7112, 9.6038)
  line L2312 (-16.7112, 9.6038) -> (-16.5545, 9.5545)
  line L2313 (-16.5545, 9.5545) -> (-16.503, 9.5433)
  line L2314 (-16.503, 9.5433) -> (-16.4584, 9.5383)
  line L2315 (-16.4584, 9.5383) -> (-16.4209, 9.5392)
  line L2316 (-16.4209, 9.5392) -> (-16.3908, 9.5457)
  line L2317 (-16.3908, 9.5457) -> (-16.3682, 9.5575)
  line L2318 (-16.3682, 9.5575) -> (-16.3534, 9.5743)
  line L2319 (-16.3534, 9.5743) -> (-16.3364, 9.6034)
  line L2320 (-16.3364, 9.6034) -> (-16.1575, 9.9013)
  line L2321 (-16.1575, 9.9013) -> (-15.9733, 10.196)
  line L2322 (-15.9733, 10.196) -> (-15.9551, 10.2244)
  line L2323 (-15.9551, 10.2244) -> (-15.9468, 10.2452)
  line L2324 (-15.9468, 10.2452) -> (-15.9466, 10.2706)
  line L2325 (-15.9466, 10.2706) -> (-15.9544, 10.3004)
  line L2326 (-15.9544, 10.3004) -> (-15.9707, 10.3342)
  line L2327 (-15.9707, 10.3342) -> (-15.9954, 10.3717)
  line L2328 (-15.9954, 10.3717) -> (-16.0287, 10.4125)
  line L2329 (-16.0287, 10.4125) -> (-16.1438, 10.5298)
  line L2330 (-16.1438, 10.5298) -> (-16.2774, 10.6739)
  line L2331 (-16.2774, 10.6739) -> (-16.4262, 10.8486)
  line L2332 (-16.4262, 10.8486) -> (-16.5875, 11.0549)
  line L2333 (-16.5875, 11.0549) -> (-16.7591, 11.2943)
  line L2334 (-16.7591, 11.2943) -> (-16.8478, 11.4265)
  line L2335 (-16.8478, 11.4265) -> (-16.9387, 11.5685)
  line L2336 (-16.9387, 11.5685) -> (-17.0299, 11.7175)
  line L2337 (-17.0299, 11.7175) -> (-17.1238, 11.8785)
  line L2338 (-17.1238, 11.8785) -> (-17.2101, 12.0338)
  arc A66 (-16.763, 12.6491) -> (-17.2101, 12.0338) centre (0, 0) ccw
  line L2339 (-16.763, 12.6491) -> (-16.5887, 12.615)
  line L2340 (-16.5887, 12.615) -> (-16.4066, 12.5755)
  line L2341 (-16.4066, 12.5755) -> (-16.2367, 12.5348)
  line L2342 (-16.2367, 12.5348) -> (-16.0735, 12.4922)
  line L2343 (-16.0735, 12.4922) -> (-15.9204, 12.4487)
  line L2344 (-15.9204, 12.4487) -> (-15.6397, 12.3595)
  line L2345 (-15.6397, 12.3595) -> (-15.3936, 12.2698)
  line L2346 (-15.3936, 12.2698) -> (-15.1815, 12.1823)
  line L2347 (-15.1815, 12.1823) -> (-15.0031, 12.0998)
  line L2348 (-15.0031, 12.0998) -> (-14.856, 12.0266)
  line L2349 (-14.856, 12.0266) -> (-14.8069, 12.0075)
  line L2350 (-14.8069, 12.0075) -> (-14.7636, 11.9956)
  line L2351 (-14.7636, 11.9956) -> (-14.7265, 11.9906)
  line L2352 (-14.7265, 11.9906) -> (-14.6957, 11.9923)
  line L2353 (-14.6957, 11.9923) -> (-14.6716, 12.0004)
  line L2354 (-14.6716, 12.0004) -> (-14.6544, 12.0147)
  line L2355 (-14.6544, 12.0147) -> (-14.633, 12.0408)
  line L2356 (-14.633, 12.0408) -> (-14.4097, 12.307)
  line L2357 (-14.4097, 12.307) -> (-14.1816, 12.5693)
  line L2358 (-14.1816, 12.5693) -> (-14.1592, 12.5944)
  line L2359 (-14.1592, 12.5944) -> (-14.1478, 12.6137)
  line L2360 (-14.1478, 12.6137) -> (-14.1436, 12.6387)
  line L2361 (-14.1436, 12.6387) -> (-14.1467, 12.6694)
  line L2362 (-14.1467, 12.6694) -> (-14.1574, 12.7053)
  line L2363 (-14.1574, 12.7053) -> (-14.1759, 12.7462)
  line L2364 (-14.1759, 12.7462) -> (-14.2025, 12.7918)
  line L2365 (-14.2025, 12.7918) -> (-14.2978, 12.9256)
  line L2366 (-14.2978, 12.9256) -> (-14.4072, 13.0888)
  line L2367 (-14.4072, 13.0888) -> (-14.5269, 13.2846)
  line L2368 (-14.5269, 13.2846) -> (-14.654, 13.5137)
  line L2369 (-14.654, 13.5137) -> (-14.786, 13.777)
  line L2370 (-14.786, 13.777) -> (-14.8529, 13.9214)
  line L2371 (-14.8529, 13.9214) -> (-14.9205, 14.0759)
  line L2372 (-14.9205, 14.0759) -> (-14.9872, 14.2373)
  line L2373 (-14.9872, 14.2373) -> (-15.0547, 14.411)
  line L2374 (-15.0547, 14.411) -> (-15.1157, 14.5779)
  arc A67 (-14.5779, 15.1157) -> (-15.1157, 14.5779) centre (0, 0) ccw
  line L2375 (-14.5779, 15.1157) -> (-14.411, 15.0547)
  line L2376 (-14.411, 15.0547) -> (-14.2373, 14.9872)
  line L2377 (-14.2373, 14.9872) -> (-14.0759, 14.9205)
  line L2378 (-14.0759, 14.9205) -> (-13.9214, 14.8528)
  line L2379 (-13.9214, 14.8528) -> (-13.777, 14.786)
  line L2380 (-13.777, 14.786) -> (-13.5137, 14.6539)
  line L2381 (-13.5137, 14.6539) -> (-13.2846, 14.5269)
  line L2382 (-13.2846, 14.5269) -> (-13.0888, 14.4072)
  line L2383 (-13.0888, 14.4072) -> (-12.9256, 14.2978)
  line L2384 (-12.9256, 14.2978) -> (-12.7918, 14.2025)
  line L2385 (-12.7918, 14.2025) -> (-12.7462, 14.1759)
  line L2386 (-12.7462, 14.1759) -> (-12.7053, 14.1574)
  line L2387 (-12.7053, 14.1574) -> (-12.6694, 14.1467)
  line L2388 (-12.6694, 14.1467) -> (-12.6387, 14.1436)
  line L2389 (-12.6387, 14.1436) -> (-12.6137, 14.1478)
  line L2390 (-12.6137, 14.1478) -> (-12.5944, 14.1592)
  line L2391 (-12.5944, 14.1592) -> (-12.5693, 14.1816)
  line L2392 (-12.5693, 14.1816) -> (-12.307, 14.4097)
  line L2393 (-12.307, 14.4097) -> (-12.0408, 14.633)
  line L2394 (-12.0408, 14.633) -> (-12.0147, 14.6544)
  line L2395 (-12.0147, 14.6544) -> (-12.0004, 14.6716)
  line L2396 (-12.0004, 14.6716) -> (-11.9923, 14.6957)
  line L2397 (-11.9923, 14.6957) -> (-11.9906, 14.7264)
  line L2398 (-11.9906, 14.7264) -> (-11.9956, 14.7636)
  line L2399 (-11.9956, 14.7636) -> (-12.0075, 14.8069)
  line L2400 (-12.0075, 14.8069) -> (-12.0266, 14.856)
  line L2401 (-12.0266, 14.856) -> (-12.0998, 15.0031)
  line L2402 (-12.0998, 15.0031) -> (-12.1823, 15.1815)
  line L2403 (-12.1823, 15.1815) -> (-12.2698, 15.3936)
  line L2404 (-12.2698, 15.3936) -> (-12.3595, 15.6397)
  line L2405 (-12.3595, 15.6397) -> (-12.4487, 15.9204)
  line L2406 (-12.4487, 15.9204) -> (-12.4922, 16.0735)
  line L2407 (-12.4922, 16.0735) -> (-12.5348, 16.2367)
  line L2408 (-12.5348, 16.2367) -> (-12.5755, 16.4066)
  line L2409 (-12.5755, 16.4066) -> (-12.615, 16.5887)
  line L2410 (-12.615, 16.5887) -> (-12.6491, 16.763)
  arc A68 (-12.0338, 17.2101) -> (-12.6491, 16.763) centre (0, 0) ccw
  line L2411 (-12.0338, 17.2101) -> (-11.8785, 17.1238)
  line L2412 (-11.8785, 17.1238) -> (-11.7175, 17.0299)
  line L2413 (-11.7175, 17.0299) -> (-11.5685, 16.9387)
  line L2414 (-11.5685, 16.9387) -> (-11.4265, 16.8478)
  line L2415 (-11.4265, 16.8478) -> (-11.2943, 16.7591)
  line L2416 (-11.2943, 16.7591) -> (-11.0549, 16.5875)
  line L2417 (-11.0549, 16.5875) -> (-10.8486, 16.4262)
  line L2418 (-10.8486, 16.4262) -> (-10.6739, 16.2774)
  line L2419 (-10.6739, 16.2774) -> (-10.5298, 16.1438)
  line L2420 (-10.5298, 16.1438) -> (-10.4125, 16.0287)
  line L2421 (-10.4125, 16.0287) -> (-10.3717, 15.9954)
  line L2422 (-10.3717, 15.9954) -> (-10.3342, 15.9707)
  line L2423 (-10.3342, 15.9707) -> (-10.3004, 15.9544)
  line L2424 (-10.3004, 15.9544) -> (-10.2706, 15.9466)
  line L2425 (-10.2706, 15.9466) -> (-10.2452, 15.9468)
  line L2426 (-10.2452, 15.9468) -> (-10.2244, 15.9551)
  line L2427 (-10.2244, 15.9551) -> (-10.196, 15.9733)
  line L2428 (-10.196, 15.9733) -> (-9.9013, 16.1575)
  line L2429 (-9.9013, 16.1575) -> (-9.6034, 16.3364)
  line L2430 (-9.6034, 16.3364) -> (-9.5743, 16.3534)
  line L2431 (-9.5743, 16.3534) -> (-9.5575, 16.3682)
  line L2432 (-9.5575, 16.3682) -> (-9.5457, 16.3908)
  line L2433 (-9.5457, 16.3908) -> (-9.5392, 16.4209)
  line L2434 (-9.5392, 16.4209) -> (-9.5383, 16.4584)
  line L2435 (-9.5383, 16.4584) -> (-9.5433, 16.503)
  line L2436 (-9.5433, 16.503) -> (-9.5545, 16.5545)
  line L2437 (-9.5545, 16.5545) -> (-9.6038, 16.7112)
  line L2438 (-9.6038, 16.7112) -> (-9.6574, 16.9003)
  line L2439 (-9.6574, 16.9003) -> (-9.7107, 17.1235)
  line L2440 (-9.7107, 17.1235) -> (-9.7608, 17.3806)
  line L2441 (-9.7608, 17.3806) -> (-9.805, 17.6718)
  line L2442 (-9.805, 17.6718) -> (-9.8239, 17.8299)
  line L2443 (-9.8239, 17.8299) -> (-9.8405, 17.9976)
  line L2444 (-9.8405, 17.9976) -> (-9.8541, 18.1718)
  line L2445 (-9.8541, 18.1718) -> (-9.8647, 18.3579)
  line L2446 (-9.8647, 18.3579) -> (-9.8711, 18.5354)
  arc A69 (-9.1934, 18.8807) -> (-9.8711, 18.5354) centre (0, 0) ccw
  line L2447 (-9.1934, 18.8807) -> (-9.0535, 18.7712)
  line L2448 (-9.0535, 18.7712) -> (-8.9092, 18.6532)
  line L2449 (-8.9092, 18.6532) -> (-8.7763, 18.5399)
  line L2450 (-8.7763, 18.5399) -> (-8.6503, 18.4279)
  line L2451 (-8.6503, 18.4279) -> (-8.5336, 18.3196)
  line L2452 (-8.5336, 18.3196) -> (-8.3239, 18.1127)
  line L2453 (-8.3239, 18.1127) -> (-8.1454, 17.921)
  line L2454 (-8.1454, 17.921) -> (-7.9961, 17.7468)
  line L2455 (-7.9961, 17.7468) -> (-7.8747, 17.5923)
  line L2456 (-7.8747, 17.5923) -> (-7.7769, 17.4603)
  line L2457 (-7.7769, 17.4603) -> (-7.7418, 17.4209)
  line L2458 (-7.7418, 17.4209) -> (-7.7086, 17.3907)
  line L2459 (-7.7086, 17.3907) -> (-7.6778, 17.3693)
  line L2460 (-7.6778, 17.3693) -> (-7.6496, 17.3569)
  line L2461 (-7.6496, 17.3569) -> (-7.6244, 17.3532)
  line L2462 (-7.6244, 17.3532) -> (-7.6026, 17.3581)
  line L2463 (-7.6026, 17.3581) -> (-7.5717, 17.3716)
  line L2464 (-7.5717, 17.3716) -> (-7.2519, 17.5075)
  line L2465 (-7.2519, 17.5075) -> (-6.9296, 17.6376)
  line L2466 (-6.9296, 17.6376) -> (-6.8982, 17.6499)
  line L2467 (-6.8982, 17.6499) -> (-6.8793, 17.6618)
  line L2468 (-6.8793, 17.6618) -> (-6.8641, 17.6822)
  line L2469 (-6.8641, 17.6822) -> (-6.853, 17.711)
  line L2470 (-6.853, 17.711) -> (-6.8462, 17.7479)
  line L2471 (-6.8462, 17.7479) -> (-6.8442, 17.7927)
  line L2472 (-6.8442, 17.7927) -> (-6.8472, 17.8453)
  line L2473 (-6.8472, 17.8453) -> (-6.8714, 18.0078)
  line L2474 (-6.8714, 18.0078) -> (-6.8947, 18.203)
  line L2475 (-6.8947, 18.203) -> (-6.9124, 18.4318)
  line L2476 (-6.9124, 18.4318) -> (-6.9217, 18.6935)
  line L2477 (-6.9217, 18.6935) -> (-6.9198, 18.9881)
  line L2478 (-6.9198, 18.9881) -> (-6.9138, 19.1471)
  line L2479 (-6.9138, 19.1471) -> (-6.9039, 19.3155)
  line L2480 (-6.9039, 19.3155) -> (-6.8901, 19.4896)
  line L2481 (-6.8901, 19.4896) -> (-6.8714, 19.675)
  line L2482 (-6.8714, 19.675) -> (-6.85, 19.8514)
  arc A70 (-6.1266, 20.0864) -> (-6.85, 19.8514) centre (0, 0) ccw
  line L2483 (-6.1266, 20.0864) -> (-6.0056, 19.9563)
  line L2484 (-6.0056, 19.9563) -> (-5.8815, 19.8173)
  line L2485 (-5.8815, 19.8173) -> (-5.7679, 19.6846)
  line L2486 (-5.7679, 19.6846) -> (-5.661, 19.5542)
  line L2487 (-5.661, 19.5542) -> (-5.5627, 19.429)
  line L2488 (-5.5627, 19.429) -> (-5.388, 19.1918)
  line L2489 (-5.388, 19.1918) -> (-5.2416, 18.9746)
  line L2490 (-5.2416, 18.9746) -> (-5.1215, 18.7791)
  line L2491 (-5.1215, 18.7791) -> (-5.0257, 18.6076)
  line L2492 (-5.0257, 18.6076) -> (-4.9497, 18.4619)
  line L2493 (-4.9497, 18.4619) -> (-4.9212, 18.4175)
  line L2494 (-4.9212, 18.4175) -> (-4.8932, 18.3824)
  line L2495 (-4.8932, 18.3824) -> (-4.8661, 18.3566)
  line L2496 (-4.8661, 18.3566) -> (-4.8402, 18.3399)
  line L2497 (-4.8402, 18.3399) -> (-4.8159, 18.3323)
  line L2498 (-4.8159, 18.3323) -> (-4.7936, 18.3337)
  line L2499 (-4.7936, 18.3337) -> (-4.761, 18.3422)
  line L2500 (-4.761, 18.3422) -> (-4.4238, 18.4264)
  line L2501 (-4.4238, 18.4264) -> (-4.0852, 18.5045)
  line L2502 (-4.0852, 18.5045) -> (-4.0522, 18.5117)
  line L2503 (-4.0522, 18.5117) -> (-4.0317, 18.5205)
  line L2504 (-4.0317, 18.5205) -> (-4.0135, 18.5383)
  line L2505 (-4.0135, 18.5383) -> (-3.998, 18.565)
  line L2506 (-3.998, 18.565) -> (-3.9856, 18.6003)
  line L2507 (-3.9856, 18.6003) -> (-3.9765, 18.6443)
  line L2508 (-3.9765, 18.6443) -> (-3.9713, 18.6968)
  line L2509 (-3.9713, 18.6968) -> (-3.9697, 18.8611)
  line L2510 (-3.9697, 18.8611) -> (-3.9623, 19.0574)
  line L2511 (-3.9623, 19.0574) -> (-3.944, 19.2862)
  line L2512 (-3.944, 19.2862) -> (-3.9122, 19.5462)
  line L2513 (-3.9122, 19.5462) -> (-3.8642, 19.8368)
  line L2514 (-3.8642, 19.8368) -> (-3.8334, 19.993)
  line L2515 (-3.8334, 19.993) -> (-3.7973, 20.1577)
  line L2516 (-3.7973, 20.1577) -> (-3.7564, 20.3275)
  line L2517 (-3.7564, 20.3275) -> (-3.7089, 20.5077)
  line L2518 (-3.7089, 20.5077) -> (-3.6602, 20.6786)
  arc A71 (-2.909, 20.7975) -> (-3.6602, 20.6786) centre (0, 0) ccw
  line L2519 (-2.909, 20.7975) -> (-2.8098, 20.6501)
  line L2520 (-2.8098, 20.6501) -> (-2.709, 20.4934)
  line L2521 (-2.709, 20.4934) -> (-2.6176, 20.3445)
  line L2522 (-2.6176, 20.3445) -> (-2.5324, 20.199)
  line L2523 (-2.5324, 20.199) -> (-2.4548, 20.06)
  line L2524 (-2.4548, 20.06) -> (-2.3194, 19.7984)
  line L2525 (-2.3194, 19.7984) -> (-2.2088, 19.561)
  line L2526 (-2.2088, 19.561) -> (-2.1207, 19.3491)
  line L2527 (-2.1207, 19.3491) -> (-2.0529, 19.1647)
  line L2528 (-2.0529, 19.1647) -> (-2.0007, 19.0089)
  line L2529 (-2.0007, 19.0089) -> (-1.9795, 18.9606)
  line L2530 (-1.9795, 18.9606) -> (-1.9573, 18.9216)
  line L2531 (-1.9573, 18.9216) -> (-1.9346, 18.8918)
  line L2532 (-1.9346, 18.8918) -> (-1.9116, 18.8712)
  line L2533 (-1.9116, 18.8712) -> (-1.8888, 18.8599)
  line L2534 (-1.8888, 18.8599) -> (-1.8665, 18.8579)
  line L2535 (-1.8665, 18.8579) -> (-1.833, 18.8612)
  line L2536 (-1.833, 18.8612) -> (-1.4868, 18.8916)
  line L2537 (-1.4868, 18.8916) -> (-1.1401, 18.9157)
  line L2538 (-1.1401, 18.9157) -> (-1.1065, 18.9177)
  line L2539 (-1.1065, 18.9177) -> (-1.0848, 18.9232)
  line L2540 (-1.0848, 18.9232) -> (-1.0641, 18.938)
  line L2541 (-1.0641, 18.938) -> (-1.0446, 18.9618)
  line L2542 (-1.0446, 18.9618) -> (-1.0268, 18.9948)
  line L2543 (-1.0268, 18.9948) -> (-1.011, 19.0368)
  line L2544 (-1.011, 19.0368) -> (-0.9976, 19.0878)
  line L2545 (-0.9976, 19.0878) -> (-0.9703, 19.2499)
  line L2546 (-0.9703, 19.2499) -> (-0.9323, 19.4426)
  line L2547 (-0.9323, 19.4426) -> (-0.8784, 19.6657)
  line L2548 (-0.8784, 19.6657) -> (-0.8063, 19.9175)
  line L2549 (-0.8063, 19.9175) -> (-0.7135, 20.1971)
  line L2550 (-0.7135, 20.1971) -> (-0.6586, 20.3465)
  line L2551 (-0.6586, 20.3465) -> (-0.5972, 20.5035)
  line L2552 (-0.5972, 20.5035) -> (-0.5302, 20.6648)
  line L2553 (-0.5302, 20.6648) -> (-0.4552, 20.8354)
  line L2554 (-0.4552, 20.8354) -> (-0.3803, 20.9966)
  arc A72 (0.3803, 20.9966) -> (-0.3803, 20.9966) centre (0, 0) ccw
  line L2555 (0.3803, 20.9966) -> (0.4552, 20.8354)
  line L2556 (0.4552, 20.8354) -> (0.5302, 20.6648)
  line L2557 (0.5302, 20.6648) -> (0.5972, 20.5035)
  line L2558 (0.5972, 20.5035) -> (0.6586, 20.3465)
  line L2559 (0.6586, 20.3465) -> (0.7135, 20.1971)
  line L2560 (0.7135, 20.1971) -> (0.8063, 19.9175)
  line L2561 (0.8063, 19.9175) -> (0.8784, 19.6657)
  line L2562 (0.8784, 19.6657) -> (0.9323, 19.4426)
  line L2563 (0.9323, 19.4426) -> (0.9703, 19.2499)
  line L2564 (0.9703, 19.2499) -> (0.9976, 19.0878)
  line L2565 (0.9976, 19.0878) -> (1.011, 19.0368)
  line L2566 (1.011, 19.0368) -> (1.0268, 18.9948)
  line L2567 (1.0268, 18.9948) -> (1.0446, 18.9618)
  line L2568 (1.0446, 18.9618) -> (1.0641, 18.938)
  line L2569 (1.0641, 18.938) -> (1.0848, 18.9232)
  line L2570 (1.0848, 18.9232) -> (1.1065, 18.9177)
  line L2571 (1.1065, 18.9177) -> (1.1401, 18.9157)
  line L2572 (1.1401, 18.9157) -> (1.4868, 18.8916)
  line L2573 (1.4868, 18.8916) -> (1.833, 18.8612)
  line L2574 (1.833, 18.8612) -> (1.8665, 18.8579)
  line L2575 (1.8665, 18.8579) -> (1.8888, 18.8599)
  line L2576 (1.8888, 18.8599) -> (1.9116, 18.8712)
  line L2577 (1.9116, 18.8712) -> (1.9346, 18.8918)
  line L2578 (1.9346, 18.8918) -> (1.9573, 18.9216)
  line L2579 (1.9573, 18.9216) -> (1.9795, 18.9606)
  line L2580 (1.9795, 18.9606) -> (2.0007, 19.0089)
  line L2581 (2.0007, 19.0089) -> (2.053, 19.1647)
  line L2582 (2.053, 19.1647) -> (2.1207, 19.3491)
  line L2583 (2.1207, 19.3491) -> (2.2088, 19.561)
  line L2584 (2.2088, 19.561) -> (2.3194, 19.7984)
  line L2585 (2.3194, 19.7984) -> (2.4548, 20.06)
  line L2586 (2.4548, 20.06) -> (2.5324, 20.199)
  line L2587 (2.5324, 20.199) -> (2.6176, 20.3445)
  line L2588 (2.6176, 20.3445) -> (2.709, 20.4934)
  line L2589 (2.709, 20.4934) -> (2.8098, 20.6501)
  line L2590 (2.8098, 20.6501) -> (2.909, 20.7975)
  arc A73 (3.6602, 20.6786) -> (2.909, 20.7975) centre (0, 0) ccw
  line L2591 (3.6602, 20.6786) -> (3.709, 20.5077)
  line L2592 (3.709, 20.5077) -> (3.7564, 20.3275)
  line L2593 (3.7564, 20.3275) -> (3.7973, 20.1577)
  line L2594 (3.7973, 20.1577) -> (3.8334, 19.993)
  line L2595 (3.8334, 19.993) -> (3.8642, 19.8368)
  line L2596 (3.8642, 19.8368) -> (3.9122, 19.5462)
  line L2597 (3.9122, 19.5462) -> (3.944, 19.2862)
  line L2598 (3.944, 19.2862) -> (3.9623, 19.0574)
  line L2599 (3.9623, 19.0574) -> (3.9697, 18.8611)
  line L2600 (3.9697, 18.8611) -> (3.9713, 18.6968)
  line L2601 (3.9713, 18.6968) -> (3.9765, 18.6443)
  line L2602 (3.9765, 18.6443) -> (3.9856, 18.6003)
  line L2603 (3.9856, 18.6003) -> (3.998, 18.565)
  line L2604 (3.998, 18.565) -> (4.0135, 18.5383)
  line L2605 (4.0135, 18.5383) -> (4.0317, 18.5205)
  line L2606 (4.0317, 18.5205) -> (4.0522, 18.5117)
  line L2607 (4.0522, 18.5117) -> (4.0852, 18.5045)
  line L2608 (4.0852, 18.5045) -> (4.4238, 18.4264)
  line L2609 (4.4238, 18.4264) -> (4.761, 18.3422)
  line L2610 (4.761, 18.3422) -> (4.7936, 18.3337)
  line L2611 (4.7936, 18.3337) -> (4.8159, 18.3323)
  line L2612 (4.8159, 18.3323) -> (4.8402, 18.3399)
  line L2613 (4.8402, 18.3399) -> (4.8661, 18.3566)
  line L2614 (4.8661, 18.3566) -> (4.8932, 18.3824)
  line L2615 (4.8932, 18.3824) -> (4.9212, 18.4175)
  line L2616 (4.9212, 18.4175) -> (4.9497, 18.4619)
  line L2617 (4.9497, 18.4619) -> (5.0257, 18.6076)
  line L2618 (5.0257, 18.6076) -> (5.1215, 18.7791)
  line L2619 (5.1215, 18.7791) -> (5.2416, 18.9746)
  line L2620 (5.2416, 18.9746) -> (5.388, 19.1918)
  line L2621 (5.388, 19.1918) -> (5.5627, 19.429)
  line L2622 (5.5627, 19.429) -> (5.661, 19.5542)
  line L2623 (5.661, 19.5542) -> (5.768, 19.6846)
  line L2624 (5.768, 19.6846) -> (5.8815, 19.8173)
  line L2625 (5.8815, 19.8173) -> (6.0056, 19.9563)
  line L2626 (6.0056, 19.9563) -> (6.1266, 20.0864)
  arc A74 (6.85, 19.8514) -> (6.1266, 20.0864) centre (0, 0) ccw
  line L2627 (6.85, 19.8514) -> (6.8714, 19.675)
  line L2628 (6.8714, 19.675) -> (6.8901, 19.4896)
  line L2629 (6.8901, 19.4896) -> (6.9039, 19.3155)
  line L2630 (6.9039, 19.3155) -> (6.9138, 19.1471)
  line L2631 (6.9138, 19.1471) -> (6.9198, 18.9881)
  line L2632 (6.9198, 18.9881) -> (6.9217, 18.6935)
  line L2633 (6.9217, 18.6935) -> (6.9124, 18.4318)
  line L2634 (6.9124, 18.4318) -> (6.8947, 18.203)
  line L2635 (6.8947, 18.203) -> (6.8714, 18.0078)
  line L2636 (6.8714, 18.0078) -> (6.8472, 17.8453)
  line L2637 (6.8472, 17.8453) -> (6.8442, 17.7927)
  line L2638 (6.8442, 17.7927) -> (6.8462, 17.7479)
  line L2639 (6.8462, 17.7479) -> (6.853, 17.711)
  line L2640 (6.853, 17.711) -> (6.8641, 17.6822)
  line L2641 (6.8641, 17.6822) -> (6.8793, 17.6618)
  line L2642 (6.8793, 17.6618) -> (6.8982, 17.6499)
  line L2643 (6.8982, 17.6499) -> (6.9296, 17.6376)
  line L2644 (6.9296, 17.6376) -> (7.2519, 17.5075)
  line L2645 (7.2519, 17.5075) -> (7.5717, 17.3716)
  line L2646 (7.5717, 17.3716) -> (7.6026, 17.3581)
  line L2647 (7.6026, 17.3581) -> (7.6244, 17.3532)
  line L2648 (7.6244, 17.3532) -> (7.6496, 17.3569)
  line L2649 (7.6496, 17.3569) -> (7.6778, 17.3693)
  line L2650 (7.6778, 17.3693) -> (7.7086, 17.3907)
  line L2651 (7.7086, 17.3907) -> (7.7418, 17.4209)
  line L2652 (7.7418, 17.4209) -> (7.7769, 17.4603)
  line L2653 (7.7769, 17.4603) -> (7.8747, 17.5923)
  line L2654 (7.8747, 17.5923) -> (7.9961, 17.7468)
  line L2655 (7.9961, 17.7468) -> (8.1454, 17.921)
  line L2656 (8.1454, 17.921) -> (8.324, 18.1127)
  line L2657 (8.324, 18.1127) -> (8.5336, 18.3196)
  line L2658 (8.5336, 18.3196) -> (8.6503, 18.4279)
  line L2659 (8.6503, 18.4279) -> (8.7763, 18.5399)
  line L2660 (8.7763, 18.5399) -> (8.9092, 18.6532)
  line L2661 (8.9092, 18.6532) -> (9.0535, 18.7712)
  line L2662 (9.0535, 18.7712) -> (9.1934, 18.8807)
  arc A75 (9.8711, 18.5354) -> (9.1934, 18.8807) centre (0, 0) ccw
  line L2663 (9.8711, 18.5354) -> (9.8647, 18.3579)
  line L2664 (9.8647, 18.3579) -> (9.8541, 18.1718)
  line L2665 (9.8541, 18.1718) -> (9.8405, 17.9976)
  line L2666 (9.8405, 17.9976) -> (9.8239, 17.8299)
  line L2667 (9.8239, 17.8299) -> (9.805, 17.6718)
  line L2668 (9.805, 17.6718) -> (9.7608, 17.3806)
  line L2669 (9.7608, 17.3806) -> (9.7107, 17.1235)
  line L2670 (9.7107, 17.1235) -> (9.6574, 16.9003)